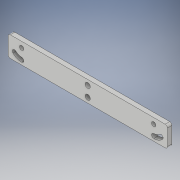
# Autodesk Inventor part: CameraBase
Saved by Autodesk Inventor 2019 (Build 230136000, 136)
## iProperties
Created: 2019-07-15
Part Number: CameraBase
Material: Generic
Document SubType Name: Modeling
Designer: aorfi
Density: 1 g/cm^3
Appearance: Default
Author: aorfi
Autodesk Inventor part; units mm, degrees
ref_plane "YZ Plane" through (0, 0, 0) normal (1, 0, 0) x (0, 1, 0)
ref_plane "XZ Plane" through (0, 0, 0) normal (0, 1, 0) x (-1, 0, 0)
ref_plane "XY Plane" through (0, 0, 0) normal (0, 0, 1) x (1, 0, 0)
sketch "Sketch1" plane through (0, 0, 0) normal (0, 0, 1) x (1, 0, 0)
  line L0 (-70, -9) -> (70, -9)
  line L1 (70, -9) -> (70, 9)
  line L2 (70, 9) -> (-70, 9)
  line L3 (-70, 9) -> (-70, -9)
  line L4 (-70, -9) -> (70, 9) construction
  line L5 (70, -9) -> (-70, 9) construction
  point P0 (0, 0)
  dimension "d3" = 18
  dimension "d26" = 140
  constraints: 12 end point, 2 midpoint, 2 parallel, 1 horizontal, 1 perpendicular
  measures "d3" distance of L2.end L0.start
  measures "d26" distance of L0.start L0.end
extrude "Extrusion1" add sketch "Sketch1" along normal mid plane 4
sketch "Sketch2" plane through (0, 0, -2) normal (0, 0, -1) x (-1, 0, 0)
  circle A0 centre (58, 4) radius 1.8986
  arc A1 (65.7065, -3.7065) -> (63.0214, -1.0214) centre (64.364, -2.364) ccw
  line L0 (64.364, -2.364) -> (58, 4) construction
  line L1 (58, 4) -> (64.364, 4) construction
  line L2 (64.364, 4) -> (64.364, -2.364) construction
  circle A2 centre (58, 4) radius 9 construction
  arc A3 (58, -3.1014) -> (58, -6.8986) centre (58, -5) ccw
  arc A4 (58, -6.8986) -> (65.7065, -3.7065) centre (58, 4) ccw
  arc A5 (58, -3.1014) -> (63.0214, -1.0214) centre (58, 4) ccw
  line L3 (70, -9) -> (70, 9) construction
  line L4 (0, -15) -> (0, 15) construction
  circle A6 centre (-58, 4) radius 1.8986
  arc A7 (-63.0214, -1.0214) -> (-65.7065, -3.7065) centre (-64.364, -2.364) ccw
  arc A8 (-58, -6.8986) -> (-58, -3.1014) centre (-58, -5) ccw
  arc A9 (-65.7065, -3.7065) -> (-58, -6.8986) centre (-58, 4) ccw
  arc A10 (-63.0214, -1.0214) -> (-58, -3.1014) centre (-58, 4) ccw
  line L5 (55.7416, 0.0884) -> (53.4833, 4) construction
  line L6 (53.4833, 4) -> (55.7416, 7.9116) construction
  line L7 (55.7416, 7.9116) -> (60.2584, 7.9116) construction
  line L8 (60.2584, 7.9116) -> (62.5167, 4) construction
  line L9 (62.5167, 4) -> (60.2584, 0.0884) construction
  line L10 (60.2584, 0.0884) -> (55.7416, 0.0884) construction
  line L11 (60.0629, -0.9851) -> (63.4076, 2.0503) construction
  line L12 (63.4076, 2.0503) -> (67.7087, 0.6715) construction
  line L13 (67.7087, 0.6715) -> (68.6651, -3.7429) construction
  line L14 (68.6651, -3.7429) -> (65.3204, -6.7783) construction
  line L15 (65.3204, -6.7783) -> (61.0193, -5.3994) construction
  line L16 (61.0193, -5.3994) -> (60.0629, -0.9851) construction
  line L17 (70, 9) -> (-70, 9) projected
  point P0 (0, 0)
  point P1 (64.364, 0.818)
  point P2 (70, 0)
  dimension "d4" = 3.7973
  dimension "d5" = 3.7973
  dimension "d6" = 45
  dimension "d7" = 3.7973
  dimension "d8" = 18
  dimension "d9" = 12
  dimension "d25" = 7.8232
  dimension "d27" = 7.8232
  dimension "d28" = 5
  constraints: 32 end point, 18 point on circle, 11 centre point, 9 symmetric about line, 6 coincident, 2 horizontal, 2 midpoint, 2 tangent, 1 perpendicular, 1 point on line, 1 vertical, 1 vertical alignment, 31 other
  measures "d4" diameter of A0
  measures "d5" diameter of A1
  measures "d6" angle of L0 L2
  measures "d7" diameter of A3
  measures "d8" diameter of A2
  measures "d9" distance from line of L0.end L3
  measures "d25" distance between parallel lines of L7 L10
  measures "d27" distance between parallel lines of L11 L14
  measures "d28" distance from line of L17 L0.end
extrude "Extrusion2" cut sketch "Sketch2" against normal through all
fillet "Fillet1" radius 2 4 edges at (-70, 9, 0) (-70, -9, 0) (70, 9, 0) (70, -9, 0)
sketch "Sketch5" plane through (0, 0, 2) normal (0, 0, 1) x (1, 0, 0)
  line L0 (0, -9) -> (0, 0) construction
  line L1 (0, 0) -> (0, 9) construction
  line L2 (68, 9) -> (-68, 9) construction
  line L3 (-68, -9) -> (68, -9) construction
  point P0 (0, -4.5)
  point P1 (0, 4.5)
  constraints: 4 end point, 4 midpoint, 1 vertical
hole "Hole2" at (0, -4.5, 2) at (0, 4.5, 2) direction (0, 0, -1) diameter 4.496 end through all clearance for "Flat Head Machine Screw (82)" size "#8" standard "Ansi Unified Screw Threads"
equation "\"d5\" = d4"
equation "\"d7\" = d4"
equation "\"d27\" = d25"
body "Solid1"
